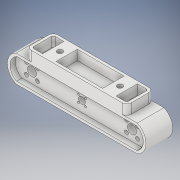
# Autodesk Inventor part: Corredera
Saved by Autodesk Inventor 2019 (Build 230136000, 136)
## iProperties
Created: 2020-04-02
Part Number: Corredera
Material: PC/ABS Plastic
Document SubType Name: Modeling
Designer: Jurgen
Density: 0.357273 g/cm^3
Appearance: White
Mass: 95.2899 g
Surface Area: 615.809 cm^2
Volume: 266.715 cm^3
Author: Jurgen
Autodesk Inventor part; units mm, degrees
ref_plane "YZ Plane" through (0, 0, 0) normal (1, 0, 0) x (0, 1, 0)
ref_plane "XZ Plane" through (0, 0, 0) normal (0, 1, 0) x (-1, 0, 0)
ref_plane "XY Plane" through (0, 0, 0) normal (0, 0, 1) x (1, 0, 0)
sketch "Sketch1" plane through (0, 0, 0) normal (0, 0, 1) x (1, 0, 0)
  circle A0 centre (75, 0) radius 15.85 construction
  circle A1 centre (66.6915, 8.3085) radius 3
  circle A2 centre (83.3085, -8.3085) radius 3
  circle A3 centre (66.6915, -8.3085) radius 3
  circle A4 centre (83.3085, 8.3085) radius 3
  circle A5 centre (75, 0) radius 6.75
  circle A6 centre (-75, 0) radius 15.85 construction
  circle A7 centre (-83.3085, 8.3085) radius 3
  circle A8 centre (-66.6915, -8.3085) radius 3
  circle A9 centre (-83.3085, -8.3085) radius 3
  circle A10 centre (-66.6915, 8.3085) radius 3
  circle A11 centre (-75, 0) radius 6.75
  circle A12 centre (5.3033, -5.3033) radius 1.5
  circle A13 centre (-5.3033, 5.3033) radius 1.5
  circle A14 centre (-5.3033, -5.3033) radius 1.5
  circle A15 centre (5.3033, 5.3033) radius 1.5
  circle A16 centre (0, 0) radius 10.75 construction
  circle A17 centre (0, 0) radius 5
  line L0 (100, -16) -> (-100, -16) construction
  line L1 (-100, -16) -> (-100, 16) construction
  line L2 (-100, 16) -> (100, 16) construction
  line L3 (100, 16) -> (100, -16) construction
  line L4 (100, -16) -> (-100, 16) construction
  line L5 (-100, -16) -> (100, 16) construction
  line L6 (0, 16) -> (-90, 16)
  line L7 (0, -16) -> (-90, -16)
  arc A18 (-90, 16) -> (-90, -16) centre (-82.2, 0) ccw
  line L8 (0, 16) -> (90, 16)
  line L9 (0, -16) -> (90, -16)
  arc A19 (90, -16) -> (90, 16) centre (82.2, 0) ccw
  point P0 (0, 0)
  point P1 (75, 0)
  point P2 (-75, 0)
  dimension "d4" = 10
  dimension "d5" = 75
  dimension "d6" = 75
  dimension "d7" = 200
  dimension "d8" = 32
  dimension "d9" = 90
  dimension "d10" = 90
  dimension "d11" = 90
  dimension "d12" = 90
  constraints: 20 centre point, 20 end point, 4 midpoint, 4 point on circle, 4 point on line, 2 parallel, 2 tangent, 1 coincident, 1 horizontal, 1 perpendicular
  measures "d4" diameter of A17
  measures "d5" distance of point (-75, 0) point (0, 0)
  measures "d6" distance of point (75, 0) point (0, 0)
  measures "d7" distance of L1.end L2.end
  measures "d8" distance of L0.end L1.end
  measures "d9" distance of L6.start L6.end
  measures "d10" distance of L7.start L7.end
  measures "d11" distance of L6.start L8.end
  measures "d12" distance of L7.start L9.end
extrude "Extrusion1" add sketch "Sketch1" along normal blind 30
sketch "Sketch2" plane through (0, 0, 0) normal (0, 0, -1) x (-1, 0, 0)
  circle A0 centre (75, 0) radius 6.75 construction
  circle A1 centre (-75, 0) radius 6.75 construction
  circle A2 centre (0, 0) radius 5 construction
  circle A3 centre (66.6915, 8.3085) radius 3 construction
  circle A4 centre (83.3085, -8.3085) radius 3 construction
  circle A5 centre (66.6915, -8.3085) radius 3 construction
  circle A6 centre (83.3085, 8.3085) radius 3 construction
  circle A7 centre (-83.3085, 8.3085) radius 3 construction
  circle A8 centre (-66.6915, -8.3085) radius 3 construction
  circle A9 centre (-83.3085, -8.3085) radius 3 construction
  circle A10 centre (-66.6915, 8.3085) radius 3 construction
  circle A11 centre (-5.3033, 5.3033) radius 1.5 construction
  circle A12 centre (5.3033, -5.3033) radius 1.5 construction
  circle A13 centre (5.3033, 5.3033) radius 1.5 construction
  circle A14 centre (-5.3033, -5.3033) radius 1.5 construction
  line L0 (-90, 16) -> (90, 16) projected
  arc A15 (-90, 16) -> (-90, -16) centre (-82.2, 0) ccw projected
  line L1 (90, -16) -> (-90, -16) projected
  arc A16 (90, -16) -> (90, 16) centre (82.2, 0) ccw projected
  line L2 (90.8741, 20) -> (-90.8741, 20)
  arc A17 (-90.8741, 20) -> (-90.8741, -20) centre (-82.2, 0) ccw
  line L3 (-90.8741, -20) -> (90.8741, -20)
  arc A18 (90.8741, -20) -> (90.8741, 20) centre (82.2, 0) ccw
  dimension "d15" = 4
  constraints: 4 end point, 4 point on circle, 2 centre point, 3 other
  measures "d15" distance between parallel lines of L0 L2
extrude "Extrusion2" add sketch "Sketch2" against normal blind 30
sketch "Sketch3" plane through (0, 0, 0) normal (0, 0, -1) x (-1, 0, 0)
  line L0 (90.8741, 20) -> (-90.8741, 20) construction
  arc A0 (-90.8741, 20) -> (-90.8741, -20) centre (-82.2, 0) ccw construction
  line L1 (-90.8741, -20) -> (90.8741, -20) construction
  arc A1 (90.8741, -20) -> (90.8741, 20) centre (82.2, 0) ccw construction
  circle A2 centre (75, 0) radius 6.75 construction
  circle A3 centre (-75, 0) radius 6.75 construction
  circle A4 centre (0, 0) radius 5 construction
  circle A5 centre (66.6915, 8.3085) radius 3 construction
  circle A6 centre (83.3085, -8.3085) radius 3 construction
  circle A7 centre (66.6915, -8.3085) radius 3 construction
  circle A8 centre (83.3085, 8.3085) radius 3 construction
  circle A9 centre (-83.3085, 8.3085) radius 3 construction
  circle A10 centre (-66.6915, -8.3085) radius 3 construction
  circle A11 centre (-83.3085, -8.3085) radius 3 construction
  circle A12 centre (-66.6915, 8.3085) radius 3 construction
  circle A13 centre (-5.3033, 5.3033) radius 1.5 construction
  circle A14 centre (5.3033, -5.3033) radius 1.5 construction
  circle A15 centre (5.3033, 5.3033) radius 1.5 construction
  circle A16 centre (-5.3033, -5.3033) radius 1.5 construction
  circle A17 centre (0, 0) radius 12
  circle A18 centre (-75, 0) radius 16.5
  circle A19 centre (75, 0) radius 16.5
  dimension "d18" = 24
  dimension "d19" = 33
  dimension "d20" = 33
  constraints: 3 centre point, 3 coincident
  measures "d18" diameter of A17
  measures "d19" diameter of A18
  measures "d20" diameter of A19
extrude "Extrusion3" cut sketch "Sketch3" against normal blind 5
sketch "Sketch4" plane through (0, 0, 30) normal (0, 0, 1) x (1, 0, 0)
  line L0 (90.8741, 20) -> (-90.8741, 20) construction
  arc A0 (-90.8741, 20) -> (-90.8741, -20) centre (-82.2, 0) ccw construction
  line L1 (-90.8741, -20) -> (90.8741, -20) construction
  arc A1 (90.8741, -20) -> (90.8741, 20) centre (82.2, 0) ccw construction
  circle A2 centre (-75, 0) radius 6.75 construction
  circle A3 centre (75, 0) radius 6.75 construction
  circle A4 centre (0, 0) radius 5 construction
  circle A5 centre (-66.6915, 8.3085) radius 3 construction
  circle A6 centre (-83.3085, -8.3085) radius 3 construction
  circle A7 centre (-66.6915, -8.3085) radius 3 construction
  circle A8 centre (-83.3085, 8.3085) radius 3 construction
  circle A9 centre (83.3085, 8.3085) radius 3 construction
  circle A10 centre (66.6915, -8.3085) radius 3 construction
  circle A11 centre (83.3085, -8.3085) radius 3 construction
  circle A12 centre (66.6915, 8.3085) radius 3 construction
  circle A13 centre (5.3033, 5.3033) radius 1.5 construction
  circle A14 centre (-5.3033, -5.3033) radius 1.5 construction
  circle A15 centre (-5.3033, 5.3033) radius 1.5 construction
  circle A16 centre (5.3033, -5.3033) radius 1.5 construction
  line L2 (90, -16) -> (-90, -16)
  arc A17 (-90, 16) -> (-90, -16) centre (-82.2, 0) ccw
  line L3 (-90, 16) -> (90, 16)
  arc A18 (90, -16) -> (90, 16) centre (82.2, 0) ccw
  dimension "d23" = 4
  constraints: 4 end point, 4 point on circle, 2 centre point, 3 other
  measures "d23" distance between parallel lines of L1 L2
extrude "Extrusion4" cut sketch "Sketch4" against normal blind 5
sketch "Sketch5" plane through (0, 0, 5) normal (0, 0, -1) x (-1, 0, 0)
  circle A0 centre (0, 0) radius 5 projected
  circle A1 centre (-5.3033, 5.3033) radius 1.5 projected
  circle A2 centre (5.3033, -5.3033) radius 1.5 projected
  circle A3 centre (5.3033, 5.3033) radius 1.5 projected
  circle A4 centre (-5.3033, -5.3033) radius 1.5 projected
  circle A5 centre (0, 0) radius 12 projected
extrude "Extrusion5" cut sketch "Sketch5" against normal blind 2
sketch "Sketch6" plane through (-75, 0, 5) normal (0, 0, -1) x (-1, 0, 0)
  circle A0 centre (0, 0) radius 6.75 projected
  circle A1 centre (-8.3085, 8.3085) radius 3 projected
  circle A2 centre (8.3085, -8.3085) radius 3 projected
  circle A3 centre (-8.3085, -8.3085) radius 3 projected
  circle A4 centre (8.3085, 8.3085) radius 3 projected
  circle A5 centre (0, 0) radius 16.5 projected
  circle A6 centre (-150, 0) radius 6.75 projected
  circle A7 centre (-158.3085, 8.3085) radius 3 projected
  circle A8 centre (-141.6915, -8.3085) radius 3 projected
  circle A9 centre (-158.3085, -8.3085) radius 3 projected
  circle A10 centre (-141.6915, 8.3085) radius 3 projected
  circle A11 centre (-150, 0) radius 16.5 projected
  point P0 (-75, 0)
extrude "Extrusion6" cut sketch "Sketch6" against normal blind 1
sketch "Sketch7" plane through (0, 0, 30) normal (0, 0, 1) x (1, 0, 0)
  arc A0 (90, -16) -> (90, 16) centre (82.2, 0) ccw projected
  line L0 (90, -16) -> (-90, -16) projected
  arc A1 (-90, 16) -> (-90, -16) centre (-82.2, 0) ccw projected
  line L1 (-90, 16) -> (90, 16) projected
  line L2 (90.8741, 20) -> (-90.8741, 20) projected
  arc A2 (-90.8741, 20) -> (-90.8741, -20) centre (-82.2, 0) ccw projected
  line L3 (-90.8741, -20) -> (90.8741, -20) projected
  arc A3 (90.8741, -20) -> (90.8741, 20) centre (82.2, 0) ccw projected
  point P0 (0, 0)
extrude "Extrusion7" add sketch "Sketch7" along normal blind 10
sketch "Sketch8" plane through (0, 0, 25) normal (0, 0, 1) x (1, 0, 0)
  circle A0 centre (-75, 0) radius 6.75 projected
  circle A1 centre (75, 0) radius 6.75 projected
  circle A2 centre (0, 0) radius 5 projected
  circle A3 centre (-66.6915, 8.3085) radius 3 projected
  circle A4 centre (-83.3085, -8.3085) radius 3 projected
  circle A5 centre (-66.6915, -8.3085) radius 3 projected
  circle A6 centre (-83.3085, 8.3085) radius 3 projected
  circle A7 centre (83.3085, 8.3085) radius 3 projected
  circle A8 centre (66.6915, -8.3085) radius 3 projected
  circle A9 centre (83.3085, -8.3085) radius 3 projected
  circle A10 centre (66.6915, 8.3085) radius 3 projected
  circle A11 centre (5.3033, 5.3033) radius 1.5 projected
  circle A12 centre (-5.3033, -5.3033) radius 1.5 projected
  circle A13 centre (-5.3033, 5.3033) radius 1.5 projected
  circle A14 centre (5.3033, -5.3033) radius 1.5 projected
  line L0 (90, -16) -> (-90, -16) projected
  arc A15 (90, -16) -> (90, 16) centre (82.2, 0) ccw projected
  line L1 (-90, 16) -> (90, 16) projected
  arc A16 (-90, 16) -> (-90, -16) centre (-82.2, 0) ccw projected
extrude "Extrusion8" add sketch "Sketch8" along normal blind 7
sketch "Sketch10" plane through (-90.8741, 20, 0) normal (0, 1, 0) x (1, 0, 0)
  circle A0 centre (135.8741, -20) radius 4
  circle A1 centre (150.8741, -20) radius 4 construction
  circle A2 centre (30.8741, -20) radius 4 construction
  circle A3 centre (45.8741, -20) radius 4
  arc A4 (15.8741, -33) -> (22.8741, -40) centre (22.8741, -33) ccw
  line L0 (22.8741, -40) -> (158.8741, -40)
  arc A5 (158.8741, -40) -> (165.8741, -33) centre (158.8741, -33) ccw
  line L1 (165.8741, -33) -> (165.8741, -7)
  arc A6 (165.8741, -7) -> (158.8741, 0) centre (158.8741, -7) ccw
  line L2 (158.8741, 0) -> (22.8741, 0)
  arc A7 (22.8741, 0) -> (15.8741, -7) centre (22.8741, -7) ccw
  line L3 (15.8741, -7) -> (15.8741, -33)
  line L4 (0, 0) -> (181.7482, 0) construction
  line L5 (0, 0) -> (0, -40) construction
  line L6 (181.7482, -40) -> (0, -40) construction
  line L7 (181.7482, 0) -> (181.7482, -40) construction
  line L8 (180.8741, -40) -> (0.8741, -40) construction
  line L9 (90.8741, -40) -> (90.8741, 0) construction
  line L10 (90.8741, 0) -> (90.8741, -40) construction
  line L11 (161.8741, -7) -> (161.8741, -33)
  arc A8 (158.8741, -36) -> (161.8741, -33) centre (158.8741, -33) ccw
  arc A9 (19.8741, -33) -> (22.8741, -36) centre (22.8741, -33) ccw
  line L12 (19.8741, -33) -> (19.8741, -7)
  arc A10 (22.8741, -4) -> (19.8741, -7) centre (22.8741, -7) ccw
  arc A11 (161.8741, -7) -> (158.8741, -4) centre (158.8741, -7) ccw
  line L13 (135.8741, -20) -> (135.8741, -36) construction
  line L14 (135.8741, -20) -> (135.8741, -4) construction
  line L15 (45.8741, -20) -> (45.8741, -36) construction
  line L16 (45.8741, -20) -> (45.8741, -4) construction
  line L17 (145.8741, -4) -> (145.8741, -36)
  line L18 (125.8741, -36) -> (125.8741, -4)
  line L19 (125.8741, -4) -> (145.8741, -36) construction
  line L20 (145.8741, -4) -> (125.8741, -36) construction
  line L21 (55.8741, -4) -> (55.8741, -36)
  line L22 (35.8741, -36) -> (35.8741, -4)
  line L23 (35.8741, -4) -> (55.8741, -36) construction
  line L24 (55.8741, -4) -> (35.8741, -36) construction
  line L25 (158.8741, -36) -> (145.8741, -36)
  line L26 (125.8741, -36) -> (55.8741, -36)
  line L27 (145.8741, -4) -> (158.8741, -4)
  line L28 (149.3741, 0) -> (149.3741, -6) projected
  line L29 (125.8741, -4) -> (55.8741, -4)
  line L30 (35.8741, -4) -> (22.8741, -4)
  line L31 (35.8741, -36) -> (22.8741, -36)
  line L32 (35.8741, -4) -> (35.8741, -36)
  line L33 (35.8741, -36) -> (22.8741, -36)
  arc A12 (19.8741, -33) -> (22.8741, -36) centre (22.8741, -33) ccw
  line L34 (19.8741, -33) -> (19.8741, -7)
  arc A13 (22.8741, -4) -> (19.8741, -7) centre (22.8741, -7) ccw
  line L35 (22.8741, -4) -> (35.8741, -4)
  point P0 (20, -7)
  dimension "d47" = 4
  dimension "d48" = 20
  dimension "d49" = 20
  constraints: 60 end point, 20 point on circle, 14 centre point, 6 midpoint, 4 parallel, 4 perpendicular, 4 point on line, 4 tangent, 3 vertical, 1 horizontal, 3 other
  measures "d47" distance between parallel lines of L1 L11
  measures "d48" distance of L18.start L17.end
  measures "d49" distance of L21.end L22.start
extrude "Extrusion11" add sketch "Sketch10" along normal blind 15
sketch "Sketch11" plane through (-45, 20, 20) normal (0, 1, 0) x (1, 0, 0)
  circle A0 centre (0, 0) radius 4 projected
  circle A1 centre (90, 0) radius 4 projected
  point P0 (45, 20)
extrude "Extrusion12" cut sketch "Sketch11" against normal blind 85
sketch "Sketch12" plane through (-90.8741, -20, 0) normal (0, -1, 0) x (1, 0, 0)
  circle A0 centre (45.8741, 20) radius 4 construction
  circle A1 centre (135.8741, 20) radius 4 construction
  line L0 (181.7482, 0) -> (0, 0) construction
  line L1 (181.7482, 0) -> (181.7482, 40) construction
  line L2 (0, 40) -> (181.7482, 40) construction
  line L3 (0, 0) -> (0, 40) construction
  line L4 (90.8741, 0) -> (90.8741, 40) construction
  line L5 (0, 0) -> (0, 40) construction
  line L6 (0, 20) -> (181.7482, 20) construction
  line L7 (145.8741, 11) -> (35.8741, 11)
  line L8 (30.8741, 16) -> (30.8741, 24)
  line L9 (35.8741, 29) -> (145.8741, 29)
  line L10 (150.8741, 24) -> (150.8741, 16)
  line L11 (150.8741, 11) -> (30.8741, 29) construction
  line L12 (30.8741, 11) -> (150.8741, 29) construction
  arc A2 (35.8741, 29) -> (30.8741, 24) centre (35.8741, 24) ccw
  arc A3 (30.8741, 16) -> (35.8741, 11) centre (35.8741, 16) ccw
  arc A4 (150.8741, 24) -> (145.8741, 29) centre (145.8741, 24) ccw
  arc A5 (145.8741, 11) -> (150.8741, 16) centre (145.8741, 16) ccw
  point P0 (90.8741, 20)
  dimension "d54" = 120
  dimension "d55" = 18
  dimension "d56" = 5
  constraints: 16 end point, 8 point on circle, 8 point on line, 8 tangent, 6 midpoint, 4 centre point, 3 equal radius, 2 parallel, 1 horizontal, 1 perpendicular
  measures "d54" distance of L11.end L12.end
  measures "d55" distance of L12.start L11.end
  measures "d56" radius of A2
extrude "Extrusion13" cut sketch "Sketch12" against normal blind 5
body "Solid1"
